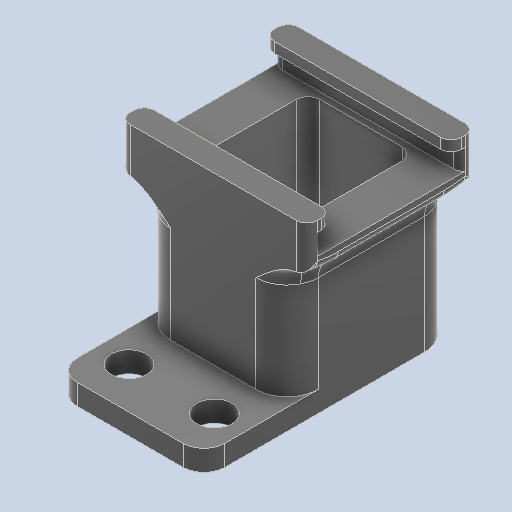
# Autodesk Inventor part: Base
Saved by Autodesk Inventor 2022 (Build 260153000, 153)
## iProperties
Created: 2021-11-22
Part Number: Base
Material: Genérico
Document SubType Name: Modeling
Designer: JK
Density: 1 g/cm^3
Appearance: Suave - Negro
Author: JK
Autodesk Inventor part; units mm, degrees
ref_plane "YZ Plane" through (0, 0, 0) normal (1, 0, 0) x (0, 1, 0)
ref_plane "XZ Plane" through (0, 0, 0) normal (0, 1, 0) x (-1, 0, 0)
ref_plane "XY Plane" through (0, 0, 0) normal (0, 0, 1) x (1, 0, 0)
sketch "Boceto1" plane through (0, 0, 0) normal (0, 1, 0) x (-1, 0, 0)
  line L0 (-7.1, 8.1) -> (7.1, 8.1)
  line L1 (7.1, 8.1) -> (7.1, -8.1)
  line L2 (7.1, -8.1) -> (-7.1, -8.1)
  line L3 (-7.1, -8.1) -> (-7.1, 8.1)
  line L4 (5.1, 6.1) -> (-5.1, 6.1)
  line L5 (-5.1, 6.1) -> (-5.1, -6.1)
  line L6 (-5.1, -6.1) -> (5.1, -6.1)
  line L7 (5.1, -6.1) -> (5.1, 6.1)
  line L8 (5.1, 6.1) -> (-5.1, -6.1) construction
  line L9 (-5.1, 6.1) -> (5.1, -6.1) construction
  point P0 (0, 0)
  point P1 (0, 0)
  point P2 (0, 0)
  point P3 (0, 0)
  point P4 (0, 0)
  point P5 (0, 0)
  dimension "d44" = 2
  dimension "d45" = 2
  dimension "d46" = 2
  dimension "d47" = 2
  dimension "d48" = 10.2
  dimension "d49" = 12.2
  constraints: 20 end point, 4 midpoint, 4 parallel, 3 coincident, 2 horizontal, 2 perpendicular
  measures "d44" distance between parallel lines of L0 L4
  measures "d45" distance between parallel lines of L2 L6
  measures "d46" distance between parallel lines of L1 L7
  measures "d47" distance between parallel lines of L3 L5
  measures "d48" distance of L4.start L4.end
  measures "d49" distance of L6.end L4.start
extrude "Extrusión1" add sketch "Boceto1" along normal blind 15
fillet "Empalme1" radius 1.15 4 edges at (5.1, 7.5, 6.1) (5.1, 7.5, -6.1) (-5.1, 7.5, -6.1) (-5.1, 7.5, 6.1)
fillet "Empalme2" radius 3 4 edges at (7.1, 7.5, -8.1) (7.1, 7.5, 8.1) (-7.1, 7.5, 8.1) (-7.1, 7.5, -8.1)
sketch "Boceto24" plane through (0, 15, 0) normal (0, 1, 0) x (1, 0, 0)
  line L0 (9, -8.1) -> (-9, -8.1)
  line L1 (-9, -8.1) -> (-9, 8.1)
  line L2 (-9, 8.1) -> (9, 8.1)
  line L3 (9, 8.1) -> (9, -8.1)
  line L4 (9, -8.1) -> (-9, 8.1) construction
  line L5 (-9, -8.1) -> (9, 8.1) construction
  line L6 (4.1, 8.1) -> (-4.1, 8.1) projected
  line L7 (-4.1, -8.1) -> (4.1, -8.1) projected
  line L8 (14.3573, -6.6) -> (-14.3573, -6.6)
  line L9 (-14.3573, -6.6) -> (-14.3573, 6.6)
  line L10 (-14.3573, 6.6) -> (14.3573, 6.6)
  line L11 (14.3573, 6.6) -> (14.3573, -6.6)
  line L12 (14.3573, -6.6) -> (-14.3573, 6.6) construction
  line L13 (-14.3573, -6.6) -> (14.3573, 6.6) construction
  arc A0 (-4.1, 8.1) -> (-7.1, 5.1) centre (-4.1, 5.1) ccw projected
  line L14 (-7.1, 5.1) -> (-7.1, -5.1) projected
  arc A1 (-7.1, -5.1) -> (-4.1, -8.1) centre (-4.1, -5.1) ccw projected
  line L15 (-4.1, -8.1) -> (4.1, -8.1) projected
  arc A2 (4.1, -8.1) -> (7.1, -5.1) centre (4.1, -5.1) ccw projected
  line L16 (7.1, -5.1) -> (7.1, 5.1) projected
  arc A3 (7.1, 5.1) -> (4.1, 8.1) centre (4.1, 5.1) ccw projected
  line L17 (4.1, 8.1) -> (-4.1, 8.1) projected
  line L18 (-5.1, -4.95) -> (-5.1, 4.95) projected
  arc A4 (-3.95, 6.1) -> (-5.1, 4.95) centre (-3.95, 4.95) ccw projected
  line L19 (-3.95, 6.1) -> (3.95, 6.1) projected
  arc A5 (5.1, 4.95) -> (3.95, 6.1) centre (3.95, 4.95) ccw projected
  line L20 (5.1, 4.95) -> (5.1, -4.95) projected
  arc A6 (3.95, -6.1) -> (5.1, -4.95) centre (3.95, -4.95) ccw projected
  line L21 (3.95, -6.1) -> (-3.95, -6.1) projected
  arc A7 (-5.1, -4.95) -> (-3.95, -6.1) centre (-3.95, -4.95) ccw projected
  point P0 (0, 0)
  point P1 (0, 0)
  point P2 (0, 0)
  point P3 (4.1, 8.1)
  point P4 (-4.1, 8.1)
  dimension "d125" = 18
  dimension "d126" = 13.2
  constraints: 24 end point, 5 midpoint, 4 parallel, 2 collinear, 2 horizontal, 2 perpendicular, 1 coincident
  measures "d125" distance of L1.end L2.end
  measures "d126" distance of L8.end L9.end
extrude "Extrusión23" add sketch "Boceto24" against normal blind 1.2 contours L0 A2 L8 L3 | L8 A2 L16 A3 L10 L3 | L0 L1 L8 A1 | L10 A3 L2 L3 | L8 L1 L10 A0 L14 A1 | L10 L1 L2 A0
sketch "Boceto25" plane through (0, 15, 0) normal (0, 1, 0) x (1, 0, 0)
  line L0 (-9, -8.1) -> (-9, 8.1) projected
  line L1 (9, -6.75) -> (-9, -6.75)
  line L2 (-9, -6.75) -> (-9, 6.75)
  line L3 (-9, 6.75) -> (9, 6.75)
  line L4 (9, 6.75) -> (9, -6.75)
  line L5 (9, -6.75) -> (-9, 6.75) construction
  line L6 (-9, -6.75) -> (9, 6.75) construction
  line L7 (-9, -8.1) -> (9, -8.1) projected
  line L8 (9, -8.1) -> (9, 8.1) projected
  line L9 (9, 8.1) -> (-9, 8.1) projected
  line L10 (-9, 8.1) -> (-9, -8.1) projected
  line L11 (-5.1, -4.95) -> (-5.1, 4.95) projected
  arc A0 (-3.95, 6.1) -> (-5.1, 4.95) centre (-3.95, 4.95) ccw projected
  line L12 (-3.95, 6.1) -> (3.95, 6.1) projected
  arc A1 (5.1, 4.95) -> (3.95, 6.1) centre (3.95, 4.95) ccw projected
  line L13 (5.1, 4.95) -> (5.1, -4.95) projected
  arc A2 (3.95, -6.1) -> (5.1, -4.95) centre (3.95, -4.95) ccw projected
  line L14 (3.95, -6.1) -> (-3.95, -6.1) projected
  arc A3 (-5.1, -4.95) -> (-3.95, -6.1) centre (-3.95, -4.95) ccw projected
  point P0 (0, 0)
  point P1 (9, 6.75)
  point P2 (9, -6.75)
  dimension "d129" = 13.5
  constraints: 12 end point, 2 midpoint, 2 parallel, 1 horizontal, 1 perpendicular, 1 point on line
  measures "d129" distance between parallel lines of L3 L1
extrude "Extrusión24" add sketch "Boceto25" along normal blind 2 contours L0 L1 L8 L7 | L0 L9 L8 L3
fillet "Empalme13" radius 2.5 6 edges at (6.2213, 13.8, 7.2213) (6.2213, 13.8, -7.2213) (7.1, 13.8, 0) (-7.1, 13.8, 0) (-6.2213, 13.8, 7.2213) (-6.2213, 13.8, -7.2213)
fillet "Empalme14" radius 1 18 edges at (-9, 15.4, -8.1) (-9, 15.4, 8.1) (-9, 13.7823, -6.8501) (-9, 13.7331, -5.6003) (-9, 13.8, -7.849) (-9, 13.7331, 5.6003) (-9, 13.7823, 6.8501) (-9, 13.8, 7.849) (-9, 13.7269, 0) (9, 15.4, 8.1) (9, 15.4, -8.1) (9, 13.7269, 0) (9, 13.7823, 6.8501) (9, 13.7331, 5.6003) (9, 13.8, 7.849) (9, 13.8, -7.849) (9, 13.7331, -5.6003) (9, 13.7823, -6.8501)
fillet "Empalme15" radius 1 4 edges at (-9, 16, 6.75) (-9, 16, -6.75) (9, 16, 6.75) (9, 16, -6.75)
sketch "Boceto26" plane through (0, 17, 0) normal (0, 1, 0) x (1, 0, 0)
  arc A0 (9, -7.1) -> (8.2401, -6.75) centre (8.2401, -7.75) ccw projected
  line L0 (8.2401, -6.75) -> (-8.2401, -6.75) projected
  arc A1 (-8.2401, -6.75) -> (-9, -7.1) centre (-8.2401, -7.75) ccw projected
  arc A2 (-9, -7.1) -> (-8, -8.1) centre (-8, -7.1) ccw projected
  line L1 (-8, -8.1) -> (8, -8.1) projected
  arc A3 (8, -8.1) -> (9, -7.1) centre (8, -7.1) ccw projected
  arc A4 (-4.1, 8.1) -> (-6.7727, 6.4625) centre (-4.1, 5.1) ccw projected
  arc A5 (8.2401, 6.75) -> (9, 7.1) centre (8.2401, 7.75) ccw projected
  arc A6 (9, 7.1) -> (8, 8.1) centre (8, 7.1) ccw projected
  line L2 (8, 8.1) -> (-8, 8.1) projected
  arc A7 (-8, 8.1) -> (-9, 7.1) centre (-8, 7.1) ccw projected
  arc A8 (-9, 7.1) -> (-8.2401, 6.75) centre (-8.2401, 7.75) ccw projected
  line L3 (-8.2401, 6.75) -> (8.2401, 6.75) projected
  line L4 (-9, 7.1) -> (-9, -7.1) projected
  line L5 (9, -7.1) -> (9, 7.1) projected
  line L6 (-9, -7.1) -> (9, -7.1)
  line L7 (9, -7.1) -> (9, -5.75)
  line L8 (9, -5.75) -> (-9, -5.75)
  line L9 (-9, -5.75) -> (-9, -7.1)
  arc A9 (9, 7.1) -> (8, 8.1) centre (8, 7.1) ccw projected
  line L10 (9, 7.1) -> (-9, 7.1)
  line L11 (-9, 7.1) -> (-9, 5.75)
  line L12 (-9, 5.75) -> (9, 5.75)
  line L13 (9, 5.75) -> (9, 7.1)
  point P0 (0, 0)
  point P1 (-9, 5.75)
  dimension "d135" = 1
  dimension "d140" = 1
  constraints: 16 end point, 4 parallel, 3 point on line, 2 horizontal, 2 perpendicular, 1 point on circle
  measures "d135" distance between parallel lines of L12 L3
  measures "d140" distance between parallel lines of L0 L8
extrude "Extrusión25" add sketch "Boceto26" along normal blind 1 contours L6 A1 L0 A0 | A0 L0 A1 L4 L8 L5 | A3 L1 A2 L6 | L12 L4 A8 L3 A5 L5 | L10 A4 L2 A6 | A5 L3 A4 L10 | L10 A7 L2 A4 | A4 L3 A8 L10
fillet "Empalme16" radius 1 4 edges at (9, 17.5, 5.75) (9, 17.5, -5.75) (-9, 17.5, 5.75) (-9, 17.5, -5.75)
sketch "Boceto27" plane through (0, 0, 0) normal (0, -1, 0) x (1, 0, 0)
  arc A0 (-7.1, -5.1) -> (-4.1, -8.1) centre (-4.1, -5.1) ccw projected
  line L0 (4.1, -8.1) -> (-4.1, -8.1) projected
  arc A1 (4.1, -8.1) -> (7.1, -5.1) centre (4.1, -5.1) ccw projected
  line L1 (7.1, 5.1) -> (7.1, -5.1) projected
  arc A2 (7.1, 5.1) -> (4.1, 8.1) centre (4.1, 5.1) ccw projected
  line L2 (-4.1, 8.1) -> (4.1, 8.1) projected
  arc A3 (-4.1, 8.1) -> (-7.1, 5.1) centre (-4.1, 5.1) ccw projected
  line L3 (-7.1, -5.1) -> (-7.1, 5.1) projected
  arc A4 (-3.95, 6.1) -> (-5.1, 4.95) centre (-3.95, 4.95) ccw projected
  line L4 (3.95, 6.1) -> (-3.95, 6.1) projected
  arc A5 (5.1, 4.95) -> (3.95, 6.1) centre (3.95, 4.95) ccw projected
  line L5 (5.1, -4.95) -> (5.1, 4.95) projected
  arc A6 (3.95, -6.1) -> (5.1, -4.95) centre (3.95, -4.95) ccw projected
  line L6 (-3.95, -6.1) -> (3.95, -6.1) projected
  arc A7 (-5.1, -4.95) -> (-3.95, -6.1) centre (-3.95, -4.95) ccw projected
  line L7 (-5.1, 4.95) -> (-5.1, -4.95) projected
  arc A8 (-6.7727, 6.4625) -> (-7.1, 5.1) centre (-4.1, 5.1) ccw projected
  line L8 (-7.1, 5.1) -> (7.1, 5.1)
  line L9 (7.1, 5.1) -> (7.1, 16.1)
  line L10 (7.1, 16.1) -> (-7.1, 16.1)
  line L11 (-7.1, 16.1) -> (-7.1, 5.1)
  line L12 (7.1, 5.1) -> (7.1, -5.1) projected
  circle A9 centre (-4.1, 12.1) radius 1.7
  circle A10 centre (4.1, 12.1) radius 1.7
  circle A11 centre (-4.1, 12.1) radius 3
  point P0 (0, 0)
  point P1 (7.1, 5.1)
  dimension "d141" = 3.4
  dimension "d142" = 3.4
  dimension "d143" = 3
  dimension "d144" = 3
  dimension "d145" = 4
  dimension "d146" = 6
  dimension "d147" = 4
  constraints: 8 end point, 3 centre point, 2 parallel, 1 coincident, 1 collinear, 1 horizontal, 1 horizontal alignment, 1 perpendicular
  measures "d141" diameter of A9
  measures "d142" diameter of A10
  measures "d143" distance from line of L11 A9.centre
  measures "d144" distance from line of L9 A10.centre
  measures "d145" distance from line of L2 A9.centre
  measures "d146" diameter of A11
  measures "d147" distance from line of A9.centre L10
extrude "Extrusión26" add sketch "Boceto27" against normal blind 2 contours A11 | L11 L10 L9 A2 L2 A3
fillet "Empalme17" radius 2 2 edges at (-7.1, 1, 16.1) (7.1, 1, 16.1)
